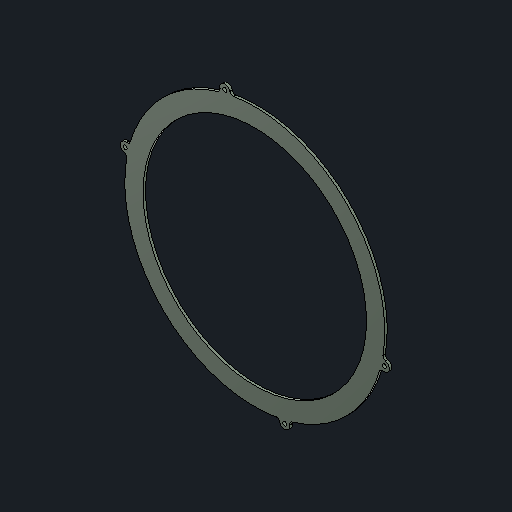
# Autodesk Inventor part: LineSensor
Saved by Autodesk Inventor 2024.2 (Build 282272000, 272)
## iProperties
Created: 2023-12-21
Part Number: LineSensor
Material: 一般
Document SubType Name: Modeling
Designer: Hanaoka
Density: 1 g/cm^3
Appearance: 既定
Author: Hanaoka
Autodesk Inventor part; units mm, degrees
ref_plane "YZ Plane" through (0, 0, 0) normal (1, 0, 0) x (0, 1, 0)
ref_plane "XZ Plane" through (0, 0, 0) normal (0, 1, 0) x (-1, 0, 0)
ref_plane "作業平面1" through (0, 0, 0) normal (0, 0, 1) x (1, 0, 0)
sketch "スケッチ1" plane through (0, 0, 0) normal (0, 0, 1) x (1, 0, 0)
  circle A0 centre (-14.624772, 63.539385) radius 64
  arc A1 (-81.893775, 52.547912) -> (-80.479561, 53.962126) centre (-81.186668, 53.255019) ccw
  line L0 (-81.893775, 52.547912) -> (-83.065348, 52.547912)
  arc A2 (-84.479561, 53.962126) -> (-83.065348, 52.547912) centre (-83.772455, 53.255019) ccw
  line L1 (-84.479561, 53.962126) -> (-84.479561, 73.133699)
  arc A3 (-83.065348, 74.547912) -> (-84.479561, 73.133699) centre (-83.772455, 73.840806) ccw
  line L2 (-83.065348, 74.547912) -> (-81.893775, 74.547912)
  arc A4 (-80.479561, 73.133699) -> (-81.893775, 74.547912) centre (-81.186668, 73.840806) ccw
  line L3 (-80.479561, 73.133699) -> (-80.479561, 53.962126)
  arc A5 (-3.479561, 132.133699) -> (-4.893775, 133.547912) centre (-4.186668, 132.840806) ccw
  line L4 (-3.479561, 132.133699) -> (-3.479561, 130.962126)
  arc A6 (-4.893775, 129.547912) -> (-3.479561, 130.962126) centre (-4.186668, 130.255019) ccw
  line L5 (-4.893775, 129.547912) -> (-24.065348, 129.547912)
  arc A7 (-25.479561, 130.962126) -> (-24.065348, 129.547912) centre (-24.772455, 130.255019) ccw
  line L6 (-25.479561, 130.962126) -> (-25.479561, 132.133699)
  arc A8 (-24.065348, 133.547912) -> (-25.479561, 132.133699) centre (-24.772455, 132.840806) ccw
  line L7 (-24.065348, 133.547912) -> (-4.893775, 133.547912)
  arc A9 (54.106225, 52.547912) -> (55.520439, 53.962126) centre (54.813332, 53.255019) ccw
  line L8 (54.106225, 52.547912) -> (52.934652, 52.547912)
  arc A10 (51.520439, 53.962126) -> (52.934652, 52.547912) centre (52.227545, 53.255019) ccw
  line L9 (51.520439, 53.962126) -> (51.520439, 73.133699)
  arc A11 (52.934652, 74.547912) -> (51.520439, 73.133699) centre (52.227545, 73.840806) ccw
  line L10 (52.934652, 74.547912) -> (54.106225, 74.547912)
  arc A12 (55.520439, 73.133699) -> (54.106225, 74.547912) centre (54.813332, 73.840806) ccw
  line L11 (55.520439, 73.133699) -> (55.520439, 53.962126)
  arc A13 (-25.479561, -5.037874) -> (-24.065348, -6.452088) centre (-24.772455, -5.744981) ccw
  line L12 (-25.479561, -5.037874) -> (-25.479561, -3.866301)
  arc A14 (-24.065348, -2.452088) -> (-25.479561, -3.866301) centre (-24.772455, -3.159194) ccw
  line L13 (-24.065348, -2.452088) -> (-4.893775, -2.452088)
  arc A15 (-3.479561, -3.866301) -> (-4.893775, -2.452088) centre (-4.186668, -3.159194) ccw
  line L14 (-3.479561, -3.866301) -> (-3.479561, -5.037874)
  arc A16 (-4.893775, -6.452088) -> (-3.479561, -5.037874) centre (-4.186668, -5.744981) ccw
  line L15 (-4.893775, -6.452088) -> (-24.065348, -6.452088)
  arc A17 (-90.380937, 104.093949) -> (-92.776199, 103.718007) centre (-91.441598, 103.033289) ccw
  arc A18 (-92.776199, 103.718007) -> (-98.248191, 90.50745) centre (-14.479561, 63.547912) ccw
  arc A19 (-98.248191, 90.50745) -> (-96.820317, 88.547912) centre (-96.820317, 90.047912) ccw
  line L16 (-96.820317, 88.547912) -> (-88.479561, 88.547912)
  arc A20 (-86.479561, 86.547912) -> (-88.479561, 88.547912) centre (-88.479561, 86.547912) ccw
  line L17 (-86.479561, 86.547912) -> (-86.479561, 40.547912)
  arc A21 (-88.479561, 38.547912) -> (-86.479561, 40.547912) centre (-88.479561, 40.547912) ccw
  line L18 (-88.479561, 38.547912) -> (-96.820317, 38.547912)
  arc A22 (-96.820317, 38.547912) -> (-98.248191, 36.588375) centre (-96.820317, 37.047912) ccw
  arc A23 (-98.248191, 36.588375) -> (-41.439099, -20.220717) centre (-14.479561, 63.547912) ccw
  arc A24 (-41.439099, -20.220717) -> (-39.479561, -18.792843) centre (-40.979561, -18.792843) ccw
  line L19 (-39.479561, -18.792843) -> (-39.479561, -10.452088)
  arc A25 (-37.479561, -8.452088) -> (-39.479561, -10.452088) centre (-37.479561, -10.452088) ccw
  line L20 (-37.479561, -8.452088) -> (8.520439, -8.452088)
  arc A26 (10.520439, -10.452088) -> (8.520439, -8.452088) centre (8.520439, -10.452088) ccw
  line L21 (10.520439, -10.452088) -> (10.520439, -18.792843)
  arc A27 (10.520439, -18.792843) -> (12.479976, -20.220717) centre (12.020439, -18.792843) ccw
  arc A28 (12.479976, -20.220717) -> (25.690533, -14.748726) centre (-14.479561, 63.547912) ccw
  arc A29 (25.690533, -14.748726) -> (26.066476, -12.353464) centre (25.005815, -13.414124) ccw
  line L22 (26.066476, -12.353464) -> (20.079693, -6.366681)
  arc A30 (20.079693, -2.124041) -> (20.079693, -6.366681) centre (22.201014, -4.245361) ccw
  line L23 (20.079693, -2.124041) -> (22.554567, 0.350833)
  arc A31 (55.435032, 28.988658) -> (51.192392, 28.988658) centre (53.313712, 26.867337) ccw
  line L24 (55.435032, 28.988658) -> (61.421815, 23.001875)
  arc A32 (61.421815, 23.001875) -> (63.817077, 23.377818) centre (62.482475, 24.062536) ccw
  arc A33 (63.817077, 23.377818) -> (69.289068, 36.588375) centre (-14.479561, 63.547912) ccw
  arc A34 (69.289068, 36.588375) -> (67.861194, 38.547912) centre (67.861194, 37.047912) ccw
  line L25 (67.861194, 38.547912) -> (59.520439, 38.547912)
  arc A35 (57.520439, 40.547912) -> (59.520439, 38.547912) centre (59.520439, 40.547912) ccw
  line L26 (57.520439, 40.547912) -> (57.520439, 86.547912)
  arc A36 (59.520439, 88.547912) -> (57.520439, 86.547912) centre (59.520439, 86.547912) ccw
  line L27 (59.520439, 88.547912) -> (67.861194, 88.547912)
  arc A37 (67.861194, 88.547912) -> (69.289068, 90.50745) centre (67.861194, 90.047912) ccw
  arc A38 (69.289068, 90.50745) -> (12.479976, 147.316542) centre (-14.479561, 63.547912) ccw
  arc A39 (12.479976, 147.316542) -> (10.520439, 145.888668) centre (12.020439, 145.888668) ccw
  line L28 (10.520439, 145.888668) -> (10.520439, 137.547912)
  arc A40 (8.520439, 135.547912) -> (10.520439, 137.547912) centre (8.520439, 137.547912) ccw
  line L29 (8.520439, 135.547912) -> (-37.479561, 135.547912)
  arc A41 (-39.479561, 137.547912) -> (-37.479561, 135.547912) centre (-37.479561, 137.547912) ccw
  line L30 (-39.479561, 137.547912) -> (-39.479561, 145.888668)
  arc A42 (-39.479561, 145.888668) -> (-41.439099, 147.316542) centre (-40.979561, 145.888668) ccw
  arc A43 (-41.439099, 147.316542) -> (-54.649656, 141.84455) centre (-14.479561, 63.547912) ccw
  arc A44 (-54.649656, 141.84455) -> (-55.025598, 139.449288) centre (-53.964938, 140.509949) ccw
  line L31 (-55.025598, 139.449288) -> (-49.038816, 133.462506)
  arc A45 (-49.038816, 129.219865) -> (-49.038816, 133.462506) centre (-51.160136, 131.341186) ccw
  line L32 (-54.342117, 123.916565) -> (-74.848214, 103.410468)
  arc A46 (-84.394155, 98.107167) -> (-80.151514, 98.107167) centre (-82.272835, 100.228487) ccw
  line L33 (-84.394155, 98.107167) -> (-90.380937, 104.093949)
  arc A47 (-32.657783, 124.912008) -> (-31.62228, 126.687656) centre (-33.083835, 126.350229) ccw
  line L34 (-31.62228, 126.687656) -> (-31.649781, 126.806774)
  arc A48 (-26.77793, 127.931529) -> (-31.649781, 126.806774) centre (-29.213855, 127.369152) ccw
  line L35 (-26.77793, 127.931529) -> (-26.75043, 127.812411)
  arc A49 (-26.75043, 127.812411) -> (-25.041333, 126.670404) centre (-25.288875, 128.149838) ccw
  arc A50 (48.642931, 52.986141) -> (-25.041333, 126.670404) centre (-14.479561, 63.547912) ccw
  arc A51 (48.642931, 52.986141) -> (49.784937, 51.277044) centre (50.122364, 52.738599) ccw
  line L36 (49.784937, 51.277044) -> (49.904056, 51.249544)
  arc A52 (48.7793, 46.377693) -> (49.904056, 51.249544) centre (49.341678, 48.813618) ccw
  line L37 (48.7793, 46.377693) -> (48.660182, 46.405194)
  arc A53 (48.660182, 46.405194) -> (46.884535, 45.369691) centre (48.322756, 44.943639) ccw
  arc A54 (3.69866, 2.183817) -> (46.884535, 45.369691) centre (-14.479561, 63.547912) ccw
  arc A55 (3.69866, 2.183817) -> (2.663157, 0.408169) centre (4.124712, 0.745596) ccw
  line L38 (2.663157, 0.408169) -> (2.690658, 0.289051)
  arc A56 (-2.181192, -0.835704) -> (2.690658, 0.289051) centre (0.254733, -0.273327) ccw
  line L39 (-2.181192, -0.835704) -> (-2.208693, -0.716586)
  arc A57 (-2.208693, -0.716586) -> (-3.91779, 0.425421) centre (-3.670248, -1.054013) ccw
  arc A58 (-77.602053, 74.109684) -> (-3.91779, 0.425421) centre (-14.479561, 63.547912) ccw
  arc A59 (-77.602053, 74.109684) -> (-78.74406, 75.818781) centre (-79.081487, 74.357226) ccw
  line L40 (-78.74406, 75.818781) -> (-78.863178, 75.846281)
  arc A60 (-77.738423, 80.718132) -> (-78.863178, 75.846281) centre (-78.300801, 78.282206) ccw
  line L41 (-77.738423, 80.718132) -> (-77.619305, 80.690631)
  arc A61 (-77.619305, 80.690631) -> (-75.843657, 81.726134) centre (-77.281878, 82.152186) ccw
  arc A62 (-32.657783, 124.912008) -> (-75.843657, 81.726134) centre (-14.479561, 63.547912) ccw
  circle A63 centre (65.069166, 92.047912) radius 2.5
  circle A64 centre (-42.979561, -16.000815) radius 2.5
  circle A65 centre (14.020439, 143.09664) radius 2.5
  circle A66 centre (-94.028289, 35.047912) radius 2.5
  circle A67 centre (49.341678, 48.813618) radius 1
  circle A68 centre (0.254733, -0.273327) radius 1
  circle A69 centre (-78.300801, 78.282206) radius 1
  circle A70 centre (-29.213855, 127.369152) radius 1
  circle A71 centre (-14.479561, 63.547912) radius 55
  circle A72 centre (19.135053, 141.074087) radius 2
  circle A73 centre (63.046613, 97.162527) radius 2
  circle A74 centre (2.020439, 127.968406) radius 2
  circle A75 centre (49.940932, 80.047912) radius 2
  line L42 (-74.848214, 103.410468) -> (-72.019786, 100.582041)
  line L43 (-71.31268, 99.874934) -> (-74.141107, 97.046507)
  line L44 (-74.848214, 97.753614) -> (-77.676641, 100.582041)
  line L45 (-49.038816, 129.219865) -> (-51.51369, 126.744992)
  line L46 (-51.51369, 126.744992) -> (-48.685263, 123.916565)
  line L47 (-47.978156, 123.209458) -> (-50.806583, 120.381031)
  line L48 (-51.51369, 121.088137) -> (-54.342117, 123.916565)
  arc A76 (-47.978156, 123.209458) -> (-48.685263, 123.916565) centre (-48.331709, 123.563011) ccw
  arc A77 (-51.51369, 121.088137) -> (-50.806583, 120.381031) centre (-51.160136, 120.734584) ccw
  arc A78 (-71.31268, 99.874934) -> (-72.019786, 100.582041) centre (-71.666233, 100.228487) ccw
  arc A79 (-74.848214, 97.753614) -> (-74.141107, 97.046507) centre (-74.49466, 97.40006) ccw
  line L49 (-77.676641, 100.582041) -> (-80.151514, 98.107167)
  line L50 (22.554567, 0.350833) -> (19.72614, 3.17926)
  arc A80 (19.019033, 3.886367) -> (19.72614, 3.17926) centre (19.372587, 3.532814) ccw
  line L51 (19.019033, 3.886367) -> (21.84746, 6.714794)
  arc A81 (22.554567, 6.007687) -> (21.84746, 6.714794) centre (22.201014, 6.361241) ccw
  line L52 (22.554567, 6.007687) -> (25.382994, 3.17926)
  line L53 (25.382994, 3.17926) -> (45.889091, 23.685357)
  line L54 (45.889091, 23.685357) -> (43.060664, 26.513784)
  arc A82 (42.353557, 27.220891) -> (43.060664, 26.513784) centre (42.70711, 26.867337) ccw
  line L55 (42.353557, 27.220891) -> (45.181984, 30.049318)
  arc A83 (45.889091, 29.342211) -> (45.181984, 30.049318) centre (45.535537, 29.695765) ccw
  line L56 (45.889091, 29.342211) -> (48.717518, 26.513784)
  line L57 (48.717518, 26.513784) -> (51.192392, 28.988658)
  point P0 (0, 0)
  dimension "d0" = 2
  dimension "d3" = 110
  constraints: 6 centre point, 5 coincident, 4 equal radius
  measures "d0" diameter of A70
  measures "d3" diameter of A71
sketch "スケッチ1 outline for 押し出し1" plane through (0, 0, 0) normal (0, 0, 1) x (1, 0, 0)
  line L0 (-78.863178, 75.846281) -> (-78.74406, 75.818781)
  arc A0 (-77.738423, 80.718132) -> (-78.863178, 75.846281) centre (-78.300801, 78.282206) ccw
  arc A1 (-78.74406, 75.818781) -> (-77.602053, 74.109684) centre (-79.081487, 74.357226) cw
  line L1 (-77.619305, 80.690631) -> (-77.738423, 80.718132)
  arc A2 (-77.602053, 74.109684) -> (-3.91779, 0.425421) centre (-14.479561, 63.547912) ccw
  arc A3 (-75.843657, 81.726134) -> (-77.619305, 80.690631) centre (-77.281878, 82.152186) cw
  arc A4 (-3.91779, 0.425421) -> (-2.208693, -0.716586) centre (-3.670248, -1.054013) cw
  arc A5 (-32.657783, 124.912008) -> (-75.843657, 81.726134) centre (-14.479561, 63.547912) ccw
  line L2 (-2.208693, -0.716586) -> (-2.181192, -0.835704)
  arc A6 (-31.62228, 126.687656) -> (-32.657783, 124.912008) centre (-33.083835, 126.350229) cw
  arc A7 (-2.181192, -0.835704) -> (2.690658, 0.289051) centre (0.254733, -0.273327) ccw
  line L3 (-31.649781, 126.806774) -> (-31.62228, 126.687656)
  line L4 (2.690658, 0.289051) -> (2.663157, 0.408169)
  arc A8 (-26.77793, 127.931529) -> (-31.649781, 126.806774) centre (-29.213855, 127.369152) ccw
  arc A9 (2.663157, 0.408169) -> (3.69866, 2.183817) centre (4.124712, 0.745596) cw
  line L5 (-26.75043, 127.812411) -> (-26.77793, 127.931529)
  arc A10 (3.69866, 2.183817) -> (46.884535, 45.369691) centre (-14.479561, 63.547912) ccw
  arc A11 (-25.041333, 126.670404) -> (-26.75043, 127.812411) centre (-25.288875, 128.149838) cw
  arc A12 (46.884535, 45.369691) -> (48.660182, 46.405194) centre (48.322756, 44.943639) cw
  arc A13 (48.642931, 52.986141) -> (-25.041333, 126.670404) centre (-14.479561, 63.547912) ccw
  line L6 (48.660182, 46.405194) -> (48.7793, 46.377693)
  arc A14 (49.784937, 51.277044) -> (48.642931, 52.986141) centre (50.122364, 52.738599) cw
  arc A15 (48.7793, 46.377693) -> (49.904056, 51.249544) centre (49.341678, 48.813618) ccw
  line L7 (49.904056, 51.249544) -> (49.784937, 51.277044)
  circle A16 centre (0.254733, -0.273327) radius 1
  circle A17 centre (-14.479561, 63.547912) radius 55
  circle A18 centre (49.341678, 48.813618) radius 1
  circle A19 centre (-78.300801, 78.282206) radius 1
  circle A20 centre (-29.213855, 127.369152) radius 1
extrude "押し出し1" add sketch "スケッチ1 outline for 押し出し1" along normal blind 1.2
